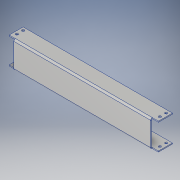
# Autodesk Inventor part: Back brace
Saved by Autodesk Inventor 2019 (Build 230136000, 136)
## iProperties
Created: 2018-11-07
Part Number: Back brace
Material: Aluminum 6061
Document SubType Name: Sheet Metal
Designer: woodk
Mass: 158.039 g
Surface Area: 596.123 cm^2
Volume: 58.533 cm^3
Density: 2.7 g/cm^3
Flat Pattern Width: 11.1699 cm
Flat Pattern Length: 30.48 cm
Flat Pattern Area: 340.459 cm^2
Sheet Metal Rule: Haakon
Sheet Metal Width: 4.398 in
Sheet Metal Length: 12.000 in
Sheet Metal Area: 52.771 in^2
Appearance: Aluminum - Flat
Author: woodk
Autodesk Inventor part; units mm, degrees
ref_plane "YZ Plane" through (0, 0, 0) normal (1, 0, 0) x (0, 1, 0)
ref_plane "XZ Plane" through (0, 0, 0) normal (0, 1, 0) x (-1, 0, 0)
ref_plane "XY Plane" through (0, 0, 0) normal (0, 0, 1) x (1, 0, 0)
sketch "Sketch1" plane through (0, 0, 0) normal (0, 0, 1) x (1, 0, 0)
  line L0 (0, 0) -> (279.4, 0)
  line L1 (279.4, 0) -> (279.4, 54.864)
  line L2 (279.4, 54.864) -> (0, 54.864)
  line L3 (0, 54.864) -> (0, 0)
  dimension "d0" = 54.864
  dimension "d1" = 279.4
  measures "d0" distance of L2.end L0.start
  measures "d1" distance of L0.start L0.end
extrude "Plate1" add sketch "Sketch1" along normal blind 2.032
sketch "Sketch2" plane through (279.4, 52.832, 2.032) normal (0, 1, 0) x (-1, 0, 0)
  line L0 (279.4, 0) -> (0, 0)
  line L1 (0, 0) -> (0, -31.75)
  line L2 (0, -31.75) -> (279.4, -31.75)
  line L3 (279.4, -31.75) -> (279.4, 0)
  constraints: 6 end point, 1 horizontal, 1 perpendicular, 1 vertical
edge flange "Flange1" height 31.75 angle 90 thickness 2.032 bend radius 1.27 thickness toward (0, 1, 0) relief tear relief width 2.032 relief depth 1.016 edges at (139.7, 54.864, 0) wall of the first edge with corners at (0, 52.832, 2.032) (279.4, 52.832, 2.032) (279.4, 52.832, -29.718) (0, 52.832, -29.718)
bend "Bend1"
corner "Corner1"
sketch "Sketch3" plane through (0, 2.032, 2.032) normal (0, -1, 0) x (1, 0, 0)
  line L0 (279.4, 0) -> (0, 0)
  line L1 (0, 0) -> (0, -31.75)
  line L2 (0, -31.75) -> (279.4, -31.75)
  line L3 (279.4, -31.75) -> (279.4, 0)
  constraints: 6 end point, 1 horizontal, 1 perpendicular, 1 vertical
edge flange "Flange2" height 31.75 angle 90 thickness 2.032 bend radius 1.27 thickness toward (0, -1, 0) relief tear relief width 2.032 relief depth 1.016 edges at (139.7, 0, 0) wall of the first edge with corners at (279.4, 2.032, 2.032) (0, 2.032, 2.032) (0, 2.032, -29.718) (279.4, 2.032, -29.718)
bend "Bend2"
corner "Corner2"
sketch "Sketch4" plane through (279.4, 52.832, -29.718) normal (1, 0, 0) x (0, 0, -1)
  line L0 (-28.448, 2.032) -> (-28.448, 0) projected
  line L1 (-28.448, 0) -> (0, 0) projected
  line L2 (0, 0) -> (0, 2.032) projected
  line L3 (0, 2.032) -> (-28.448, 2.032) projected
  arc A0 (-28.448, 2.032) -> (-31.75, -1.27) centre (-28.448, -1.27) ccw projected
  line L4 (-29.718, -1.27) -> (-31.75, -1.27) projected
  arc A1 (-28.448, 0) -> (-29.718, -1.27) centre (-28.448, -1.27) ccw projected
  line L5 (-28.448, -50.8) -> (-28.448, -52.832) projected
  line L6 (-28.448, -52.832) -> (0, -52.832) projected
  line L7 (0, -50.8) -> (0, -52.832) projected
  line L8 (-28.448, -50.8) -> (0, -50.8) projected
  arc A2 (-29.718, -49.53) -> (-28.448, -50.8) centre (-28.448, -49.53) ccw projected
  line L9 (-31.75, -49.53) -> (-29.718, -49.53) projected
  arc A3 (-31.75, -49.53) -> (-28.448, -52.832) centre (-28.448, -49.53) ccw projected
  point P0 (-29.718, -52.832)
extrude "Extrusion1" add sketch "Sketch4" along normal blind 12.7 contours L3 L2 L1 L0 | L8 L7 L6 L5
sketch "Sketch5" plane through (0, 52.832, -29.718) normal (-1, 0, 0) x (0, 0, 1)
  line L0 (28.448, 0) -> (28.448, 2.032) projected
  line L1 (28.448, 2.032) -> (0, 2.032) projected
  line L2 (0, 0) -> (0, 2.032) projected
  line L3 (28.448, 0) -> (0, 0) projected
  arc A0 (29.718, -1.27) -> (28.448, 0) centre (28.448, -1.27) ccw projected
  line L4 (31.75, -1.27) -> (29.718, -1.27) projected
  arc A1 (31.75, -1.27) -> (28.448, 2.032) centre (28.448, -1.27) ccw projected
  line L5 (28.448, -52.832) -> (28.448, -50.8) projected
  line L6 (28.448, -50.8) -> (0, -50.8) projected
  line L7 (0, -50.8) -> (0, -52.832) projected
  line L8 (0, -52.832) -> (28.448, -52.832) projected
  arc A2 (28.448, -52.832) -> (31.75, -49.53) centre (28.448, -49.53) ccw projected
  line L9 (29.718, -49.53) -> (31.75, -49.53) projected
  arc A3 (28.448, -50.8) -> (29.718, -49.53) centre (28.448, -49.53) ccw projected
  point P0 (29.718, -52.832)
extrude "Extrusion2" add sketch "Sketch5" along normal blind 12.7 contours L3 L2 L1 L0 | L8 L7 L6 L5
sketch "Sketch6" plane through (279.4, 54.864, -1.27) normal (0, 1, 0) x (1, 0, 0)
  line L0 (0, -3.302) -> (-279.4, -3.302) projected
  line L1 (12.7, 28.448) -> (12.7, 0) projected
  line L2 (-292.1, 0) -> (-292.1, 28.448) projected
  point P0 (-279.4, -1.27)
  point P1 (6.35, 9.398)
  point P2 (6.35, 22.098)
  point P3 (-285.75, 9.398)
  point P4 (-285.75, 22.098)
  dimension "d27" = 12.7
  dimension "d28" = 12.7
  dimension "d29" = 6.35
  dimension "d30" = 6.35
  constraints: 2 horizontal alignment, 2 vertical alignment
  measures "d27" distance of point (6.35, 9.398) point (6.35, 22.098)
  measures "d28" distance from line of L0 point (6.35, 9.398)
  measures "d29" distance from line of L1 point (6.35, 22.098)
  measures "d30" distance from line of L2 point (-285.75, 22.098)
hole "Hole1" at (285.75, 54.864, -10.668) at (285.75, 54.864, -23.368) at (-6.35, 54.864, -10.668) at (-6.35, 54.864, -23.368) direction (0, -1, 0) diameter 4.9784 end through all
equation "\"d36\" = Thickness"
equation "\"d2\" = Thickness"
equation "\"d3\" = BendReliefWidth"
equation "\"d4\" = BendReliefDepth"
equation "\"d5\" = MinimumRemnant"
equation "\"d6\" = TransitionRadius"
equation "\"d9\" = BendRadius"
equation "\"d10\" = CornerReliefSize"
equation "\"d11\" = GapSize"
equation "\"d12\" = JacobiRadiusSize"
equation "\"d13\" = BendReliefWidth"
equation "\"d14\" = BendReliefDepth"
equation "\"d15\" = MinimumRemnant"
equation "\"d16\" = TransitionRadius"
equation "\"d19\" = BendRadius"
equation "\"d20\" = CornerReliefSize"
equation "\"d21\" = GapSize"
equation "\"d22\" = JacobiRadiusSize"
equation "\"BendReliefWidth\" = Thickness"
equation "\"BendReliefDepth\" = 0.5 * Thickness"
equation "\"CornerReliefSize\" = 4 * Thickness"
equation "\"MinimumRemnant\" = 2 * Thickness"
equation "\"TransitionRadius\" = BendRadius"
equation "\"JacobiRadiusSize\" = BendRadius"
equation "\"GapSize\" = Thickness"
equation "\"Thickness\" = 2.032"
equation "\"BendRadius\" = 1.27"
body "Solid1"
